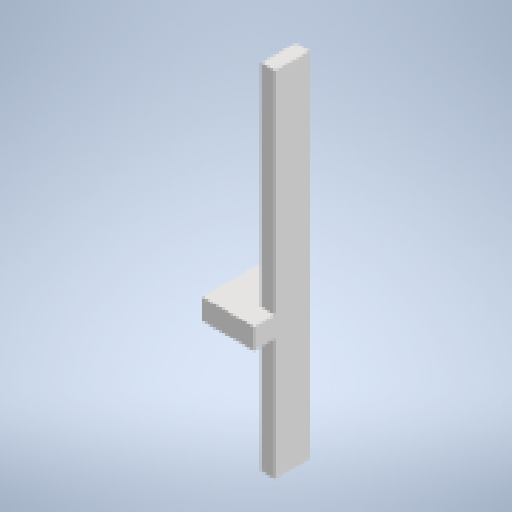
# Autodesk Inventor part: Part2
Saved by Autodesk Inventor 2024.2 (Build 282272000, 272)
## iProperties
Created: 2024-04-08
Part Number: Part2
Material: Generic
Document SubType Name: Modeling
Designer: admin
Density: 1 g/cm^3
Appearance: Default
Author: admin
Autodesk Inventor part; units mm, degrees
ref_plane "YZ Plane" through (0, 0, 0) normal (1, 0, 0) x (0, 1, 0)
ref_plane "XZ Plane" through (0, 0, 0) normal (0, 1, 0) x (-1, 0, 0)
ref_plane "XY Plane" through (0, 0, 0) normal (0, 0, 1) x (1, 0, 0)
sketch "Sketch1" plane through (0, 0, 0) normal (0, 0, 1) x (1, 0, 0)
  line L0 (-750, 300) -> (750, 300)
  line L1 (750, 300) -> (750, -300)
  line L2 (750, -300) -> (-750, -300)
  line L3 (-750, -300) -> (-750, 300)
  line L4 (-750, 300) -> (750, -300) construction
  line L5 (750, 300) -> (-750, -300) construction
  point P0 (0, 0)
  dimension "d0" = 1500
  dimension "d1" = 600
  constraints: 12 end point, 2 midpoint, 2 parallel, 1 horizontal, 1 perpendicular
  measures "d0" distance of L1.end L2.end
  measures "d1" distance of L0.end L1.end
extrude "Extrusion1" add sketch "Sketch1" along normal blind 1600
sketch "Sketch2" plane through (0, 0, 0) normal (0, 0, 1) x (1, 0, 0)
  line L0 (-750, -300) -> (750, -300) projected
  line L1 (750, -300) -> (750, 300) projected
  line L2 (750, 300) -> (-750, 300) projected
  line L3 (-750, 300) -> (-750, -300) projected
  line L4 (750, 300) -> (350, 300)
  line L5 (350, 300) -> (350, 6400)
  line L6 (350, 6400) -> (750, 6400)
  line L7 (750, 6400) -> (750, 300)
  line L8 (-750, -300) -> (750, -300) projected
  line L9 (750, -300) -> (350, -300)
  line L10 (350, -300) -> (350, -3800)
  line L11 (350, -3800) -> (750, -3800)
  line L12 (750, -3800) -> (750, -300)
  point P0 (0, 0)
  dimension "d4" = 400
  dimension "d5" = 6100
  dimension "d6" = 3500
  constraints: 16 end point, 4 parallel, 2 horizontal, 2 perpendicular, 1 collinear
  measures "d4" distance of L5.end L6.end
  measures "d5" distance of L4.end L5.end
  measures "d6" distance of L10.end L9.end
extrude "Extrusion2" add sketch "Sketch2" along normal blind 1000 contours L0 L12 L11 L10 | L5 L6 L7 L2
body "Solid1"
